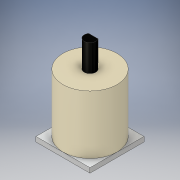
# Autodesk Inventor part: 2804S_NEMA2115_1Gearbox
Saved by Autodesk Inventor 2019.4 (Build 234330000, 330)
## iProperties
Created: 2021-02-01
Part Number: 2804S_NEMA2115_1Gearbox
Material: Generic
Document SubType Name: Modeling
Designer: Jorian Brusind
Density: 1 g/cm^3
Appearance: Default
Author: Jorian Brusind
Autodesk Inventor part; units mm, degrees
ref_plane "YZ Plane" through (0, 0, 0) normal (1, 0, 0) x (0, 1, 0)
ref_plane "XZ Plane" through (0, 0, 0) normal (0, 1, 0) x (-1, 0, 0)
ref_plane "XY Plane" through (0, 0, 0) normal (0, 0, 1) x (1, 0, 0)
sketch "Sketch1" plane through (0, 0, 0) normal (0, 1, 0) x (-1, 0, 0)
  line L0 (0, 0) -> (56.4, 0)
  line L1 (56.4, 0) -> (56.4, -56.4)
  line L2 (56.4, -56.4) -> (0, -56.4)
  line L3 (0, -56.4) -> (0, 0)
  dimension "d0" = 56.4
  dimension "d1" = 56.4
  constraints: 8 end point, 2 parallel, 1 horizontal, 1 perpendicular
  measures "d0" distance of L1.end L2.end
  measures "d1" distance of L0.end L1.end
extrude "Extrusion1" add sketch "Sketch1" along normal blind 5
sketch "Sketch2" plane through (0, 5, 0) normal (0, 1, 0) x (1, 0, 0)
  circle A0 centre (-28.2, 28.2) radius 28.2
  line L0 (-56.4, 0) -> (0, 0) projected
  line L1 (-56.4, 56.4) -> (-56.4, 0) projected
  dimension "d4" = 56.4
  dimension "d5" = 28.2
  dimension "d6" = 28.2
  constraints: 1 centre point
  measures "d4" diameter of A0
  measures "d5" distance from line of L0 A0.centre
  measures "d6" distance from line of L1 A0.centre
extrude "Extrusion2" add sketch "Sketch2" along normal blind 61 contours A0
sketch "Sketch3" plane through (-28.2, 66, -28.2) normal (0, 1, 0) x (1, 0, 0)
  arc A0 (0, 28.2) -> (-28.2, 0) centre (0, 0) ccw projected
  circle A1 centre (0, 0) radius 6
  point P0 (28.2, -28.2)
  dimension "d9" = 12
  constraints: 1 centre point, 1 coincident
  measures "d9" diameter of A1
extrude "g" add sketch "Sketch3" along normal blind 28
sketch "Sketch4" plane through (-28.2, 94, -28.2) normal (0, 1, 0) x (1, 0, 0)
  circle A0 centre (0, 0) radius 6 projected
  line L0 (0, 0) -> (0, -6)
  line L1 (0, 0) -> (0, 3.5)
  line L2 (0, 3.5) -> (-5, 3.5)
  line L3 (0, 3.5) -> (5, 3.5)
  line L4 (5, 3.5) -> (-5, 3.5)
  line L5 (-5, 3.5) -> (-5, 8.5)
  line L6 (-5, 8.5) -> (5, 8.5)
  line L7 (5, 8.5) -> (5, 3.5)
  point P0 (28.2, -28.2)
  dimension "d12" = 3.5
  dimension "d13" = 5
  dimension "d14" = 5
  dimension "d15" = 10
  dimension "d16" = 5
  constraints: 16 end point, 3 horizontal, 2 parallel, 1 perpendicular, 1 point on line, 1 vertical, 1 vertical alignment, 1 other
  measures "d12" distance of L0.start L1.end
  measures "d13" distance of L1.end L2.end
  measures "d14" distance of L1.end L3.end
  measures "d15" distance of L5.end L6.end
  measures "d16" distance of L4.end L5.end
extrude "Extrusion4" cut sketch "Sketch4" against normal blind 22 contours L2 L5 L6 L7 L3 A0 | A0 L3 L2
sketch "Sketch5" plane through (0, 0, 0) normal (0, -1, 0) x (1, 0, 0)
  circle A0 centre (-28.2, -28.2) radius 28.2 projected
  circle A1 centre (-28.2, -28.2) radius 4
  point P0 (0, 0)
  dimension "d19" = 8
  constraints: 1 centre point, 1 coincident
  measures "d19" diameter of A1
extrude "Extrusion5" cut sketch "Sketch5" against normal blind 20 contours A1
body "Solid1"
